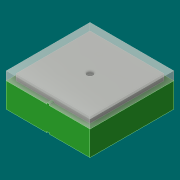
# Autodesk Inventor part: 13360-30xxVE
Saved by Autodesk Inventor 2016 (Build 200138000, 138)
## iProperties
Created: 2016-06-07
Part Number: 13360-30xxVE
Material: ABS Plastic
Document SubType Name: Modeling
Designer: sawaiz
Density: 1.06 g/cm^3
Appearance: Smooth - White
Author: sawaiz
Autodesk Inventor part; units mm, degrees
ref_plane "YZ Plane" through (0, 0, 0) normal (1, 0, 0) x (0, 1, 0)
ref_plane "XZ Plane" through (0, 0, 0) normal (0, 1, 0) x (-1, 0, 0)
ref_plane "XY Plane" through (0, 0, 0) normal (0, 0, 1) x (1, 0, 0)
sketch "Sketch1" plane through (0, 0, 0) normal (0, 1, 0) x (-1, 0, 0)
  line L0 (1.7, 1.7) -> (-1.7, 1.7)
  line L1 (-1.7, 1.7) -> (-1.7, -1.7)
  line L2 (-1.7, -1.7) -> (1.7, -1.7)
  line L3 (1.7, -1.7) -> (1.7, 1.7)
  line L4 (1.7, 1.7) -> (-1.7, -1.7) construction
  line L5 (-1.7, 1.7) -> (1.7, -1.7) construction
  point P0 (0, 0)
  dimension "d0" = 3.4
  dimension "d1" = 3.4
  constraints: 12 end point, 2 midpoint, 2 parallel, 1 horizontal, 1 perpendicular
  measures "d0" distance of L2.end L1.end
  measures "d1" distance of L1.end L0.end
extrude "Extrusion1" add sketch "Sketch1" along normal blind 1
sketch "Sketch2" plane through (0, 1, 0) normal (0, 1, 0) x (1, 0, 0)
  line L0 (1.5, -1.5) -> (-1.5, -1.5)
  line L1 (-1.5, -1.5) -> (-1.5, 1.5)
  line L2 (-1.5, 1.5) -> (1.5, 1.5)
  line L3 (1.5, 1.5) -> (1.5, -1.5)
  line L4 (1.5, -1.5) -> (-1.5, 1.5) construction
  line L5 (-1.5, -1.5) -> (1.5, 1.5) construction
  point P0 (0, 0)
  dimension "d4" = 3
  dimension "d5" = 3
  constraints: 12 end point, 2 midpoint, 2 parallel, 1 horizontal, 1 perpendicular
  measures "d4" distance of L1.end L2.end
  measures "d5" distance of L0.end L1.end
extrude "Extrusion2" add sketch "Sketch2" along normal blind 0.25 separate body
sketch "Sketch8" plane through (0, 1, 0) normal (0, 1, 0) x (1, 0, 0)
  line L0 (-1.7, -1.7) -> (1.7, -1.7) projected
  line L1 (1.7, -1.7) -> (1.7, 1.7) projected
  line L2 (1.7, 1.7) -> (-1.7, 1.7) projected
  line L3 (-1.7, 1.7) -> (-1.7, -1.7) projected
  line L4 (-1.5, -1.5) -> (1.5, -1.5) projected
  line L5 (-0.05, -1.7) -> (0.05, -1.7)
  line L6 (0.05, -1.7) -> (0.05, -1.5)
  line L7 (0.05, -1.5) -> (-0.05, -1.5)
  line L8 (-0.05, -1.5) -> (-0.05, -1.7)
  point P0 (0, 0)
  point P1 (0, -1.5)
  dimension "d35" = 0.1
  dimension "d36" = 0.05
  constraints: 8 end point, 2 parallel, 2 point on line, 1 horizontal, 1 midpoint, 1 perpendicular
  measures "d35" distance between parallel lines of L8 L6
  measures "d36" distance from line of L6 point (0, -1.5)
extrude "Extrusion6" add sketch "Sketch8" along normal blind 0.05 contours L8 L4 L6 L0 bodies 1
sketch "Sketch3" plane through (0, 1, 0) normal (0, 1, 0) x (1, 0, 0)
  line L0 (-1.7, -1.7) -> (-0.05, -1.7) projected
  line L1 (1.7, -1.7) -> (1.7, 1.7) projected
  line L2 (1.7, 1.7) -> (-1.7, 1.7) projected
  line L3 (-1.7, 1.7) -> (-1.7, -1.7) projected
  line L4 (-1.5, -1.5) -> (1.5, -1.5) projected
  line L5 (1.5, -1.5) -> (1.5, 1.5) projected
  line L6 (1.5, 1.5) -> (-1.5, 1.5) projected
  line L7 (-1.5, 1.5) -> (-1.5, -1.5) projected
  line L8 (0.05, -1.5) -> (0.05, -1.7) projected
  line L9 (0.05, -1.7) -> (1.7, -1.7) projected
  line L10 (-0.05, -1.7) -> (-0.05, -1.5) projected
  line L11 (-0.05, -1.5) -> (0.05, -1.5) projected
  point P0 (0, 0)
extrude "Extrusion3" add sketch "Sketch3" along normal blind 0.35 separate body contours L3 L2 L1 L9 L8 L4 L5 L6 L7 L10 L0
sketch "Sketch9" plane through (0, 1.05, 0) normal (0, 1, 0) x (1, 0, 0)
  point P0 (0, 0)
sketch "Sketch10" plane through (0, 1.35, 0) normal (0, 1, 0) x (1, 0, 0)
  line L0 (-0.05, -1.7) -> (0.05, -1.7) projected
  line L1 (0.05, -1.7) -> (0.05, -1.5) projected
  line L2 (0.05, -1.5) -> (-0.05, -1.5) projected
  line L3 (-0.05, -1.5) -> (-0.05, -1.7) projected
  point P0 (0, 0)
extrude "Extrusion7" add sketch "Sketch10" against normal up to surface (0.3 mm away) bodies 3
sketch "Sketch5" plane through (0, 1.25, 0) normal (0, 1, 0) x (1, 0, 0)
  point P0 (0, 0)
  point P1 (0, 0)
  constraints: 1 coincident
hole "Hole1" at (0, 1.25, 0) direction (0, -1, 0) diameter 0.254 depth 0.1 tip angle 118 bodies 2
sketch "Sketch4" plane through (0, 1.35, 0) normal (0, 1, 0) x (1, 0, 0)
  line L0 (-1.5, -1.5) -> (-1.5, 1.5) projected
  line L1 (-1.5, 1.5) -> (1.5, 1.5) projected
  line L2 (1.5, 1.5) -> (1.5, -1.5) projected
  line L3 (1.5, -1.5) -> (-1.5, -1.5) projected
  line L4 (1.7, -1.7) -> (1.7, 1.7) projected
  line L5 (1.7, 1.7) -> (-1.7, 1.7) projected
  line L6 (-1.7, 1.7) -> (-1.7, -1.7) projected
  line L7 (-1.7, -1.7) -> (1.7, -1.7) projected
  point P0 (0, 0)
extrude "Extrusion4" add sketch "Sketch4" against normal up to surface (0.1 mm away) contours L0 L1 L2 L3 bodies 3
sketch "Sketch6" plane through (0, 0, 0) normal (0, -1, 0) x (1, 0, 0)
  circle A0 centre (0, 0) radius 0.127 projected
  line L0 (1.1, 1.1) -> (-1.1, 1.1)
  line L1 (-1.1, 1.1) -> (-1.1, -1.1)
  line L2 (-1.1, -1.1) -> (1.1, -1.1)
  line L3 (1.1, -1.1) -> (1.1, 1.1)
  line L4 (1.1, 1.1) -> (-1.1, -1.1) construction
  line L5 (-1.1, 1.1) -> (1.1, -1.1) construction
  dimension "d19" = 2.2
  dimension "d20" = 2.2
  constraints: 12 end point, 4 coincident, 2 midpoint, 2 parallel, 1 horizontal, 1 perpendicular
  measures "d19" distance of L2.end L1.end
  measures "d20" distance of L1.end L0.end
hole "Hole2" at (0, 0, 0) at (1.1, 0, -1.1) at (-1.1, 0, -1.1) at (-1.1, 0, 1.1) at (1.1, 0, 1.1) direction (0, 1, 0) diameter 0.8 depth 0.05 bodies 1
sketch "Sketch7" plane through (0, 0.05, 0) normal (0, -1, 0) x (1, 0, 0)
  circle A0 centre (0, 0) radius 0.4 projected
  circle A1 centre (1.1, -1.1) radius 0.4 projected
  circle A2 centre (-1.1, -1.1) radius 0.4 projected
  circle A3 centre (-1.1, 1.1) radius 0.4 projected
  circle A4 centre (1.1, 1.1) radius 0.4 projected
  circle A5 centre (1.1, -1.1) radius 0.35
  circle A6 centre (-1.1, -1.1) radius 0.4 projected
  circle A7 centre (-1.1, -1.1) radius 0.35
  circle A8 centre (-1.1, 1.1) radius 0.35
  circle A9 centre (1.1, 1.1) radius 0.35
  circle A10 centre (0, 0) radius 0.35
  dimension "d28" = 0.7
  dimension "d29" = 0.7
  dimension "d30" = 0.7
  dimension "d31" = 0.7
  dimension "d32" = 0.7
  constraints: 5 centre point, 5 coincident
  measures "d28" diameter of A5
  measures "d29" diameter of A7
  measures "d30" diameter of A8
  measures "d31" diameter of A9
  measures "d32" diameter of A10
extrude "Extrusion5" add sketch "Sketch7" along normal blind 0.05 separate body contours A5 | A7 | A8 | A9 | A10
sketch "Sketch11" plane through (0, 0, 0) normal (0, -1, 0) x (1, 0, 0)
  circle A0 centre (-1.1, 1.1) radius 0.4 projected
  circle A1 centre (1.1, -1.1) radius 0.4 projected
  circle A2 centre (0, 0) radius 0.4 projected
  circle A3 centre (-1.1, -1.1) radius 0.4 projected
  circle A4 centre (1.1, 1.1) radius 0.4 projected
  line L0 (-1.7, 1.7) -> (1.7, 1.7) projected
  line L1 (-1.7, -1.7) -> (-1.7, 1.7) projected
  line L2 (1.7, -1.7) -> (-1.7, -1.7) projected
  line L3 (1.7, 1.7) -> (1.7, -1.7) projected
  line L4 (-0.05, 1.7) -> (0.05, 1.7)
  line L5 (0.05, 1.7) -> (0.05, 1.5)
  line L6 (0.05, 1.5) -> (-0.05, 1.5)
  line L7 (-0.05, 1.5) -> (-0.05, 1.7)
  point P0 (0, 1.7)
  dimension "d41" = 0.1
  dimension "d42" = 0.2
  dimension "d43" = 0.05
  constraints: 8 end point, 2 parallel, 1 horizontal, 1 midpoint, 1 perpendicular, 1 point on line
  measures "d41" distance of L5.end L6.end
  measures "d42" distance of L4.end L5.end
  measures "d43" distance from line of L5 point (0, 1.7)
extrude "Extrusion8" cut sketch "Sketch11" against normal blind 0.05 contours L0 L5 L6 L7 bodies 1
body "Solid1"
body "Solid2"
body "Solid3"
body "Solid4"
